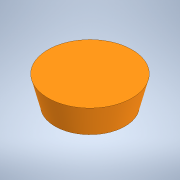
# Autodesk Inventor part: crucible
Saved by Autodesk Inventor 2020 (Build 240168000, 168)
## iProperties
RuleStatus: InUse
Created: 2026-01-29
Part Number: crucible
Material: Concrete
Document SubType Name: Modeling
Designer: Furikake
Density: 2.40731 g/cm^3
Appearance: Orange
Author: Furikake
Autodesk Inventor part; units mm, degrees
ref_plane "YZ Plane" through (0, 0, 0) normal (1, 0, 0) x (0, 1, 0)
ref_plane "XZ Plane" through (0, 0, 0) normal (0, 1, 0) x (-1, 0, 0)
ref_plane "XY Plane" through (0, 0, 0) normal (0, 0, 1) x (1, 0, 0)
sketch "Sketch1" plane through (0, 0, 0) normal (0, 0, 1) x (1, 0, 0)
  line L0 (0, 40) -> (0, -40)
  line L1 (0, 40) -> (120, 40)
  line L2 (120, 40) -> (100, -40)
  line L3 (100, -40) -> (0, -40)
  point P0 (0, 0)
  point P1 (0, 0)
  point P2 (0, -520)
  dimension "d1" = 80
  dimension "d8" = 120
  dimension "d9" = 100
  constraints: 8 end point, 2 horizontal, 1 coincident, 1 midpoint, 1 point on line, 1 vertical
  measures "d1" distance of L0.start L0.end
  measures "d8" distance of L0.start L1.end
  measures "d9" distance of L2.end L0.end
revolve "Revolution1" add sketch "Sketch1" angle 360 about axis through (0, 40, 0) along (0, -1, 0)
equation "\"d1\" = crucibleSupThickness"
equation "\"d8\" = crucibleSupTopRadius"
equation "\"d9\" = crucibleSupBottomRadius"
equation "\"crucibleSupBottomRadius\" = 100"
equation "\"crucibleSupThickness\" = 80"
equation "\"crucibleSupTopRadius\" = 120"
body "Solid1"
